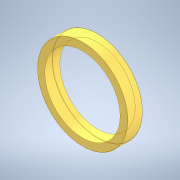
# Autodesk Inventor part: reifen
Saved by Autodesk Inventor 2022 (Build 260153000, 153)
## iProperties
Created: 2022-11-16
Part Number: reifen
Material: Polyurethan-Kautschuk Polurea 60
Document SubType Name: Modeling
Designer: Friedrich Walmrath
Density: 0.94464 g/cm^3
Appearance: Polyurethan-Kautschuk Polurea 60
Mass: 8.154 g
Surface Area: 51.3936 cm^2
Volume: 8.63186 cm^3
Author: Friedrich Walmrath
Autodesk Inventor part; units mm, degrees
ref_plane "YZ Plane" through (0, 0, 0) normal (1, 0, 0) x (0, 1, 0)
ref_plane "XZ Plane" through (0, 0, 0) normal (0, 1, 0) x (-1, 0, 0)
ref_plane "XY Plane" through (0, 0, 0) normal (0, 0, 1) x (1, 0, 0)
sketch "Skizze1" plane through (0, 0, 0) normal (0, 0, 1) x (1, 0, 0)
  circle A0 centre (0, 0) radius 30
  circle A1 centre (0, 0) radius 25
  dimension "d0" = 60
  dimension "d1" = 50
  constraints: 2 centre point, 2 coincident
  measures "d0" diameter of A0
  measures "d1" diameter of A1
extrude "Extrusion1" add sketch "Skizze1" along normal blind 10
chamfer "Fase1" distance 0.2 angle 45 2 edges at (-30, 0, 10) (-30, 0, 0)
